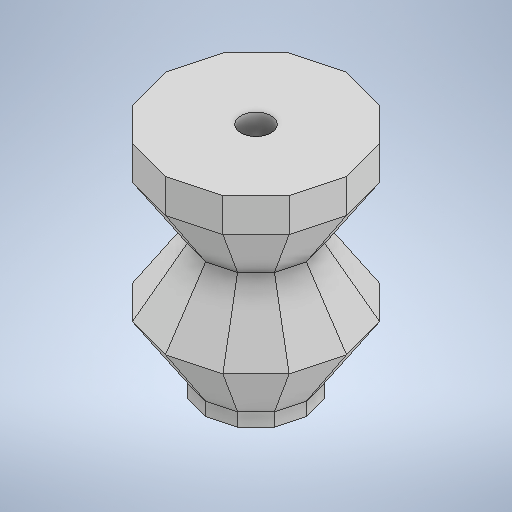
# Autodesk Inventor part: diameter27
Saved by Autodesk Inventor 2025.1 (Build 291241000, 241)
## iProperties
Created: 2024-08-09
Part Number: diameter27
Material: 일반
Document SubType Name: Modeling
Designer: 82103
Density: 1 g/cm^3
Appearance: 기본값
Author: 82103
Autodesk Inventor part; units mm, degrees
ref_plane "YZ Plane" through (0, 0, 0) normal (1, 0, 0) x (0, 1, 0)
ref_plane "XY Plane" through (0, 0, 0) normal (0, 0, 1) x (1, 0, 0)
sketch "스케치1" plane through (0, 0, 0) normal (0, 1, 0) x (-1, 0, 0)
  line L0 (11.6913, 6.75) -> (13.5, 0)
  line L1 (13.5, 0) -> (11.6913, -6.75)
  line L2 (11.6913, -6.75) -> (6.75, -11.6913)
  line L3 (6.75, -11.6913) -> (0, -13.5)
  line L4 (0, -13.5) -> (-6.75, -11.6913)
  line L5 (-6.75, -11.6913) -> (-11.6913, -6.75)
  line L6 (-11.6913, -6.75) -> (-13.5, 0)
  line L7 (-13.5, 0) -> (-11.6913, 6.75)
  line L8 (-11.6913, 6.75) -> (-6.75, 11.6913)
  line L9 (-6.75, 11.6913) -> (0, 13.5)
  line L10 (0, 13.5) -> (6.75, 11.6913)
  line L11 (6.75, 11.6913) -> (11.6913, 6.75)
  point P0 (0, 0)
  point P1 (0, 0)
  dimension "d0" = 27
  constraints: 24 end point, 1 coincident, 1 vertical alignment, 25 other
  measures "d0" distance of L6.end L0.end
ref_plane "작업 평면1" through (0, 9, 0) normal (0, 1, 0) x (-1, 0, 0)
sketch "스케치2" plane through (0, 9, 0) normal (0, 1, 0) x (-1, 0, 0)
  line L0 (3.75, -6.4952) -> (0, -7.5)
  line L1 (0, -7.5) -> (-3.75, -6.4952)
  line L2 (-3.75, -6.4952) -> (-6.4952, -3.75)
  line L3 (-6.4952, -3.75) -> (-7.5, 0)
  line L4 (-7.5, 0) -> (-6.4952, 3.75)
  line L5 (-6.4952, 3.75) -> (-3.75, 6.4952)
  line L6 (-3.75, 6.4952) -> (0, 7.5)
  line L7 (0, 7.5) -> (3.75, 6.4952)
  line L8 (3.75, 6.4952) -> (6.4952, 3.75)
  line L9 (6.4952, 3.75) -> (7.5, 0)
  line L10 (7.5, 0) -> (6.4952, -3.75)
  line L11 (6.4952, -3.75) -> (3.75, -6.4952)
  point P0 (0, 0)
  point P1 (0, 0)
  dimension "d2" = 15
  constraints: 24 end point, 1 coincident, 1 horizontal alignment, 25 other
  measures "d2" distance of L3.end L9.end
loft "로프트1" add profiles "스케치2", "스케치1"
mirror "미러1" about plane through (0, 9, 0) normal (0, 1, 0) of "로프트1"
mirror "미러2" about plane through (0, 0, 0) normal (0, 1, 0) of "로프트1"
shell "쉘1" thickness 0.5 removed faces 0 ; own thickness 2 on faces at (-8.5377, -1.5, 8.5377) (-3.125, -1.5, 11.6627) (3.125, -1.5, 11.6627) (8.5377, -1.5, 8.5377) (11.6627, -1.5, 3.125) (11.6627, -1.5, -3.125) (8.5377, -1.5, -8.5377) (3.125, -1.5, -11.6627) (-3.125, -1.5, -11.6627) (-8.5377, -1.5, -8.5377) (-11.6627, -1.5, -3.125) (-11.6627, -1.5, 3.125) (-11.6627, 16.5, -3.125) (-11.6627, 16.5, 3.125) (-8.5377, 16.5, 8.5377) (-8.5377, 16.5, -8.5377) (-3.125, 16.5, -11.6627) (-3.125, 16.5, 11.6627) (3.125, 16.5, 11.6627) (8.5377, 16.5, 8.5377) (11.6627, 16.5, 3.125) (11.6627, 16.5, -3.125) (8.5377, 16.5, -8.5377) (3.125, 16.5, -11.6627)
sketch "스케치3" plane through (-3.75, -9, -6.4952) normal (0, -1, 0) x (0.9659258, 0, -0.258819)
  line L0 (0, 0) -> (3.8823, 0) projected
  line L1 (3.8823, 0) -> (7.2444, 1.9411) projected
  line L2 (7.2444, 1.9411) -> (9.1856, 5.3033) projected
  line L3 (9.1856, 5.3033) -> (9.1856, 9.1856) projected
  line L4 (9.1856, 9.1856) -> (7.2444, 12.5477) projected
  line L5 (7.2444, 12.5477) -> (3.8823, 14.4889) projected
  line L6 (3.8823, 14.4889) -> (0, 14.4889) projected
  line L7 (0, 14.4889) -> (-3.3622, 12.5477) projected
  line L8 (-3.3622, 12.5477) -> (-5.3033, 9.1856) projected
  line L9 (-5.3033, 9.1856) -> (-5.3033, 5.3033) projected
  line L10 (-5.3033, 5.3033) -> (-3.3622, 1.9411) projected
  line L11 (-3.3622, 1.9411) -> (0, 0) projected
  point P0 (1.9411, 7.2444)
extrude "돌출1" add sketch "스케치3" along normal blind 2
sketch "스케치4" plane through (-6.75, 18, -11.6913) normal (0, 1, 0) x (0.9659258, 0, -0.258819)
  line L0 (0, 0) -> (6.9881, 0) projected
  line L1 (-6.0519, -3.4941) -> (0, 0) projected
  line L2 (-9.5459, -9.5459) -> (-6.0519, -3.4941) projected
  line L3 (-9.5459, -16.5341) -> (-9.5459, -9.5459) projected
  line L4 (-6.0519, -22.5859) -> (-9.5459, -16.5341) projected
  line L5 (0, -26.08) -> (-6.0519, -22.5859) projected
  line L6 (6.9881, -26.08) -> (0, -26.08) projected
  line L7 (13.04, -22.5859) -> (6.9881, -26.08) projected
  line L8 (16.5341, -16.5341) -> (13.04, -22.5859) projected
  line L9 (16.5341, -9.5459) -> (16.5341, -16.5341) projected
  line L10 (13.04, -3.4941) -> (16.5341, -9.5459) projected
  line L11 (6.9881, 0) -> (13.04, -3.4941) projected
  point P0 (3.4941, -13.04)
extrude "돌출2" add sketch "스케치4" along normal blind 5
sketch "스케치5" plane through (-6.75, 23, -11.6913) normal (0, 1, 0) x (0.9659258, 0, -0.258819)
  circle A0 centre (3.4941, -13.04) radius 2.25
  dimension "d13" = 4.5
  constraints: 1 centre point, 1 coincident
  measures "d13" diameter of A0
extrude "돌출3" cut sketch "스케치5" against normal blind 5.5
